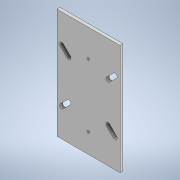
# Autodesk Inventor part: gateGasket
Saved by Autodesk Inventor 2021.2 (Build 252289000, 289)
## iProperties
Created: 2020-11-21
Part Number: gateGasket
Material: Generic
Document SubType Name: Modeling
Designer: robst
Density: 1 g/cm^3
Appearance: Default
Author: robst
Autodesk Inventor part; units mm, degrees
ref_plane "YZ Plane" through (0, 0, 0) normal (1, 0, 0) x (0, 1, 0)
ref_plane "XZ Plane" through (0, 0, 0) normal (0, 1, 0) x (-1, 0, 0)
ref_plane "XY Plane" through (0, 0, 0) normal (0, 0, 1) x (1, 0, 0)
sketch "Sketch2" plane through (0, 0, 0) normal (0, 0, 1) x (1, 0, 0)
  line L0 (-50.8, -88.9) -> (50.8, -88.9)
  line L1 (50.8, -88.9) -> (50.8, 88.9)
  line L2 (50.8, 88.9) -> (-50.8, 88.9)
  line L3 (-50.8, 88.9) -> (-50.8, -88.9)
  line L4 (-50.8, -88.9) -> (50.8, 88.9) construction
  line L5 (50.8, -88.9) -> (-50.8, 88.9) construction
  point P0 (0, 0)
  dimension "d0" = 101.6
  dimension "d1" = 177.8
  constraints: 12 end point, 2 midpoint, 2 parallel, 1 horizontal, 1 perpendicular
  measures "d0" distance of L2.end L1.end
  measures "d1" distance of L1.end L0.end
extrude "Extrusion1" add sketch "Sketch2" against normal blind 4.7625
sketch "Sketch3" plane through (0, 0, 0) normal (0, 0, 1) x (1, 0, 0)
  line L0 (50.8, 88.9) -> (50.8, -88.9) construction
  line L1 (-50.8, -50.8) -> (50.8, -50.8) construction
  line L2 (50.8, -50.8) -> (50.8, 50.8) construction
  line L3 (50.8, 50.8) -> (-50.8, 50.8) construction
  line L4 (-50.8, 50.8) -> (-50.8, -50.8) construction
  line L5 (-50.8, -50.8) -> (50.8, 50.8) construction
  line L6 (50.8, -50.8) -> (-50.8, 50.8) construction
  line L7 (50.8, 88.9) -> (-50.8, 88.9) construction
  line L8 (-42.9423, 42.9423) -> (-31.717, 31.717) construction
  line L9 (-45.331, 40.5535) -> (-34.1057, 29.3282)
  line L10 (-29.3282, 34.1057) -> (-40.5535, 45.331)
  arc A0 (-40.5535, 45.331) -> (-45.331, 40.5535) centre (-42.9423, 42.9423) ccw
  arc A1 (-34.1057, 29.3282) -> (-29.3282, 34.1057) centre (-31.717, 31.717) ccw
  line L11 (-34.1057, -29.3282) -> (-45.331, -40.5535)
  arc A2 (-45.331, -40.5535) -> (-40.5535, -45.331) centre (-42.9423, -42.9423) ccw
  line L12 (-40.5535, -45.331) -> (-29.3282, -34.1057)
  arc A3 (-29.3282, -34.1057) -> (-34.1057, -29.3282) centre (-31.717, -31.717) ccw
  line L13 (29.3282, -34.1057) -> (40.5535, -45.331)
  arc A4 (40.5535, -45.331) -> (45.331, -40.5535) centre (42.9423, -42.9423) ccw
  line L14 (45.331, -40.5535) -> (34.1057, -29.3282)
  arc A5 (34.1057, -29.3282) -> (29.3282, -34.1057) centre (31.717, -31.717) ccw
  line L15 (34.1057, 29.3282) -> (45.331, 40.5535)
  arc A6 (45.331, 40.5535) -> (40.5535, 45.331) centre (42.9423, 42.9423) ccw
  line L16 (40.5535, 45.331) -> (29.3282, 34.1057)
  arc A7 (29.3282, 34.1057) -> (34.1057, 29.3282) centre (31.717, 31.717) ccw
  point P0 (0, 0)
  point P1 (0, 0)
  point P2 (-37.3296, 37.3296)
  dimension "d4" = 38.1
  dimension "d5" = 101.6
  dimension "d6" = 6.7564
  dimension "d7" = 19.05
  dimension "d8" = 15.875
  dimension "d13" = 360
  constraints: 32 end point, 16 point on circle, 8 centre point, 4 tangent, 3 midpoint, 3 parallel, 3 point on line, 1 horizontal, 1 perpendicular, 41 other
  measures "d4" distance between parallel lines of L3 L7
  measures "d5" distance between parallel lines of L1 L3
  measures "d6" distance between parallel lines of L9 L10
  measures "d7" distance of point (-37.33, 37.33) L3.end
  measures "d8" distance of L8.end L8.start
extrude "Extrusion3" cut sketch "Sketch3" against normal through all
sketch "Sketch4" plane through (0, 0, 0) normal (0, 0, 1) x (1, 0, 0)
  line L0 (50.8, 88.9) -> (-50.8, 88.9) construction
  line L1 (0, 88.9) -> (0, -88.9) construction
  line L2 (-50.8, -88.9) -> (50.8, -88.9) construction
  point P0 (0, 0)
  point P1 (0, 44.45)
  point P2 (0, -57.15)
  dimension "d17" = 44.45
  dimension "d18" = 101.6
  constraints: 2 end point, 2 midpoint, 2 point on line
  measures "d17" distance from line of point (0, 44.45) L0
  measures "d18" distance of point (0, -57.15) point (0, 44.45)
hole "Hole1" at (0, 44.45, 0) at (0, -57.15, 0) direction (0, 0, -1) diameter 3.6576 end through all clearance for "Flat Head Machine Screw (82)" size "#6" standard "Ansi Unified Screw Threads"
body "Solid1"
